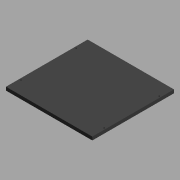
# Autodesk Inventor part: box_top
Saved by Autodesk Inventor 2019 (Build 230136000, 136)
## iProperties
Part Number: box_top
Material: Generic
Document SubType Name: Modeling
Designer: Javi
Appearance: Default
Author: Javi
Autodesk Inventor part; units mm, degrees
ref_plane "YZ Plane" through (0, 0, 0) normal (1, 0, 0) x (0, 1, 0)
ref_plane "XZ Plane" through (0, 0, 0) normal (0, 1, 0) x (-1, 0, 0)
ref_plane "XY Plane" through (0, 0, 0) normal (0, 0, 1) x (1, 0, 0)
sketch "Sketch1" plane through (0, 0, 0) normal (0, 1, 0) x (-1, 0, 0)
  line L0 (0, 0) -> (-260, 0)
  line L1 (-260, 0) -> (-260, -246)
  line L2 (-260, -246) -> (0, -246)
  line L3 (0, -246) -> (0, 0)
  dimension "d0" = 260
  dimension "d1" = 246
  constraints: 8 end point, 2 parallel, 1 horizontal, 1 perpendicular
  measures "d0" distance of L2.end L1.end
  measures "d1" distance of L1.end L0.end
extrude "Extrusion1" add sketch "Sketch1" along normal blind 10
sketch "Sketch2" plane through (0, 10, 0) normal (0, 1, 0) x (1, 0, 0)
  circle A0 centre (5, 206) radius 2
  line L0 (0, 246) -> (0, 0) projected
  line L1 (260, 246) -> (0, 246) projected
  circle A1 centre (255, 206) radius 2
  circle A2 centre (5, 40) radius 2
  circle A3 centre (255, 40) radius 2
  dimension "d4" = 4
  dimension "d5" = 5
  dimension "d6" = 40
  dimension "d9" = 250
  dimension "d12" = 166
  constraints: 4 centre point, 1 horizontal, 1 vertical, 6 other
  measures "d4" diameter of A0
  measures "d5" distance from line of L0 A0.centre
  measures "d6" distance from line of L1 A0.centre
  measures "d9" distance of A0.centre A1.centre
  measures "d12" distance of A0.centre A2.centre
extrude "Extrusion2" cut sketch "Sketch2" against normal through all
equation "\"d4\" = screws"
equation "\"screws\" = 4"
body "Solid1"
